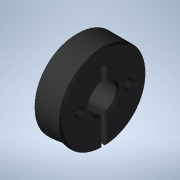
# Autodesk Inventor part: SCSWA8-8b
Saved by Autodesk Inventor 2021 (Build 250183000, 183)
## iProperties
Created: 2025-04-08
Part Number: SCSWA8-8b
Material: Generic
Catalog Web Link: www.cadenas.de
Description: SCSW, PSCSW, SSCSW, SCSWA, SCSWAW-b-Set Collars - Slit 2 Hole/2 Tap - Standard Type - 2 Tap Type
Vendor: MISUMI
Document SubType Name: Modeling
Designer: psAdmin
Manufacturer: MISUMI
Mass: 3.06754 g
Surface Area: 20.419 cm^2
Volume: 3.06754 cm^3
Density: 1 g/cm^3
Appearance: PSOLRGB-175-175-175
Category: PARTsolutions
Company: MISUMI
Title: SCSWA8-8b
Author: Cadenas PARTsolutions
Comments: Set Collars - Slit 2 Hole/2 Tap - Standard Type - 2 Tap Type
PSOL_IDENT_0: {$CADENAS_DATA/23d-libs/misumi/metric/03_set_collars/scsw_b.prj},198 {VTYP=3D},{NB=SCSWA8-8b},{LINA=
PSOL_IDENT_1: SCSWA8-8b},{NN=SCSW, PSCSW, SSCSW, SCSWA, SCSWAW-b},{DATE=29.11.2024 04:05:21},{GEOMDATE=15.09.2021
PSOL_IDENT_2: 06:01:21},{VERSION=},{LINEID=50},{WBVAR=MAT,ST,BS},{WBNUMERIC=BS}  {NB=SCSWA8-8b},{LINA=SCSWA8-8b},{
PSOL_IDENT_3: KT=DUMMY},{PN=SCSWA8-8},{TYPE=SCSWA},{MAT=2017},{MATA='1045','S45C Equivalent','304','SUS304 Equival
PSOL_IDENT_4: ent','2017','2017 Aluminum Alloy'},{ST=-},{AC=Hexagon Socket Head Set Screw 1 Pc. (304 Stainless Ste
PSOL_IDENT_5: el) },{D=8},{BS=8},{B1=8,10,12},{D1=25},{M=M3},{THMD=3},{THDMIN=2.459},{ST0='-','-','Clear Anodize','
PSOL_IDENT_6: Clear Anodize'},{DD=3.4},{R=3.00},{W=1.5},{X=8.0},{Y=5.0},{Z=7~9},{S=3.5},{P=14},{C=0.5},{L=10},{M1=
PSOL_IDENT_7: M3},{ZZ=8},{THMD1=3},{THDMIN1=2.459}
NB: SCSWA8-8b
NN: SCSW, PSCSW, SSCSW, SCSWA, SCSWAW-b
NT: Set Collars - Slit 2 Hole/2 Tap - Standard Type - 2 Tap Type
NBSYN: $PN.b
LINA: SCSWA8-8b
CATALOG: Misumi
PN: SCSWA8-8
MAT: 2017 Aluminum Alloy
ST: -
AC: Hexagon Socket Head Set Screw 1 Pc. (304 Stainless Steel)
D: 8
BS: 8
D1: 25
M: M3
DD: 3.4
R: 3
W: 1.5
X: 8
Y: 5
Z: 7~9
S: 3.5
P: 14
M1: M3
SUPPLIER: MISUMI
ARTICLENO: SCSWA8-8b
BOMINFO: SCSWA8-8b
CREATOR: CADENAS GmbH
Autodesk Inventor part; units mm, degrees
sketch "Sketch_1" plane through (0, 0, 0) normal (0, 0, 1) x (1, 0, 0)
  line L0 (4, 0) -> (-4, 0)
  line L1 (-4, 12) -> (-4, 4.5)
  line L2 (-4, 4.5) -> (-3.5, 4)
  line L3 (-3.5, 4) -> (3.5, 4)
  line L4 (3.5, 4) -> (4, 4.5)
  line L5 (4, 4.5) -> (4, 12)
  line L6 (4, 12) -> (3.5, 12.5)
  line L7 (3.5, 12.5) -> (-3.5, 12.5)
  line L8 (-3.5, 12.5) -> (-4, 12)
  constraints: 18 end point
revolve "Revolution1" add sketch "Sketch_1" angle 360 about axis through (4, 0, 0) along (1, 0, 0)
sketch "Sketch_2" plane through (0, 0, 0) normal (1, 0, 0) x (0, 1, 0)
  line L0 (-12.5, 0.75) -> (-12.5, -0.75)
  line L1 (-12.5, -0.75) -> (8, -0.75)
  line L2 (8, -0.75) -> (8, 0.75)
  line L3 (8, 0.75) -> (-12.5, 0.75)
  constraints: 8 end point
extrude "Extrusion1" cut sketch "Sketch_2" along normal mid plane 8
sketch "Sketch_3" plane through (0, 0, 0) normal (1, 0, 0) x (0, 1, 0)
  line L0 (-8, 12.5) -> (-8, 0)
  line L1 (-8, 0) -> (-9.7, 0)
  line L2 (-9.7, 0) -> (-9.7, 5)
  line L3 (-9.7, 5) -> (-11, 5)
  line L4 (-11, 5) -> (-11, 12.5)
  line L5 (-11, 12.5) -> (-8, 12.5)
  line L6 (-8, 12.5) -> (-8, 0)
  constraints: 14 end point
revolve "Revolution2" cut sketch "Sketch_3" angle 360 about axis through (0, -8, 12.5) along (0, 0, 1)
sketch "Sketch_4" plane through (0, 0, 0) normal (1, 0, 0) x (0, 1, 0)
  line L0 (-8, -12.75) -> (-8, -0.75)
  line L1 (-8, -0.75) -> (-6.5, -0.75)
  line L2 (-6.5, -0.75) -> (-6.7705, -1.0205)
  line L3 (-6.7705, -1.0205) -> (-6.7705, -12.75)
  line L4 (-6.7705, -12.75) -> (-8, -12.75)
  line L5 (-8, -12.75) -> (-8, -0.75)
  constraints: 12 end point
revolve "Revolution3" cut sketch "Sketch_4" angle 360 about axis through (0, -8, -12.75) along (0, 0, -1)
thread "Thread1" size "M3x0.5" class "6H" standard "ISO Metric profile" length 9.6566
sketch "Sketch_7" plane through (0, 0, -7) normal (0, 0, 1) x (1, 0, 0)
  line L0 (4, 0) -> (-4, 0)
  line L1 (-4, 0) -> (-4, 1.5)
  line L2 (-4, 1.5) -> (-3.7295, 1.2295)
  line L3 (-3.7295, 1.2295) -> (3.7295, 1.2295)
  line L4 (3.7295, 1.2295) -> (4, 1.5)
  line L5 (4, 1.5) -> (4, 0)
  line L6 (4, 0) -> (-4, 0)
  constraints: 14 end point
revolve "Revolution4" cut sketch "Sketch_7" angle 360 about axis through (4, 0, -7) along (1, 0, 0)
thread "Thread2" size "M3x0.5" class "6H" standard "ISO Metric profile" full length
sketch "Sketch_8" plane through (0, 0, 7) normal (0, 0, 1) x (1, 0, 0)
  line L0 (4, 0) -> (-4, 0)
  line L1 (-4, 0) -> (-4, 1.5)
  line L2 (-4, 1.5) -> (-3.7295, 1.2295)
  line L3 (-3.7295, 1.2295) -> (3.7295, 1.2295)
  line L4 (3.7295, 1.2295) -> (4, 1.5)
  line L5 (4, 1.5) -> (4, 0)
  line L6 (4, 0) -> (-4, 0)
  constraints: 14 end point
revolve "Revolution5" cut sketch "Sketch_8" angle 360 about axis through (4, 0, 7) along (1, 0, 0)
thread "Thread3" size "M3x0.5" class "6H" standard "ISO Metric profile" full length
ref_plane "body_screw_XY" through (0, -8, 5) normal (0, 0, 1) x (1, 0, 0)
ref_plane "body_screw_YZ" through (0, -8, 5) normal (1, 0, 0) x (0, 1, 0)
ref_plane "body_screw_ZX" through (0, -8, 5) normal (0, 1, 0) x (0, 0, 1)
body "Solid1"
